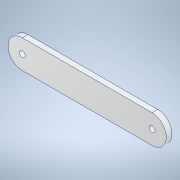
# Autodesk Inventor part: オムニ_支え板横
Saved by Autodesk Inventor 2021 (Build 250183000, 183)
## iProperties
Created: 2022-02-03
Part Number: オムニ_支え板横
Material: アルミニウム 6061
Document SubType Name: Modeling
Designer: hirohumi
Density: 2.7 g/cm^3
Appearance: アルミニウム - フラット
Author: hirohumi
Autodesk Inventor part; units mm, degrees
ref_plane "YZ Plane" through (0, 0, 0) normal (1, 0, 0) x (0, 1, 0)
ref_plane "XZ Plane" through (0, 0, 0) normal (0, 1, 0) x (-1, 0, 0)
ref_plane "XY Plane" through (0, 0, 0) normal (0, 0, 1) x (1, 0, 0)
sketch "スケッチ1" plane through (0, 0, 0) normal (0, 0, 1) x (1, 0, 0)
  circle A0 centre (-34.269, 0) radius 1.6
  circle A1 centre (34.269, 0) radius 1.6
  arc A2 (-34.269, 7.5) -> (-34.269, -7.5) centre (-34.269, 0) ccw
  arc A3 (34.269, -7.5) -> (34.269, 7.5) centre (34.269, 0) ccw
  line L0 (-34.269, 7.5) -> (34.269, 7.5)
  line L1 (-34.269, -7.5) -> (34.269, -7.5)
  point P0 (0, 0)
  dimension "d0" = 3.2
  dimension "d1" = 3.2
  dimension "d2" = 68.538
  dimension "d3" = 34.269
  dimension "d6" = 7.5
  constraints: 4 centre point, 4 end point, 4 point on circle, 4 tangent, 2 coincident, 2 horizontal alignment, 1 horizontal
  measures "d0" diameter of A0
  measures "d1" diameter of A1
  measures "d2" distance of A1.centre A0.centre
  measures "d3" distance of point (0, 0) A0.centre
  measures "d6" radius of A2
extrude "押し出し1" add sketch "スケッチ1" along normal blind 3
equation "\"d3\" = 0.5 * d2"
